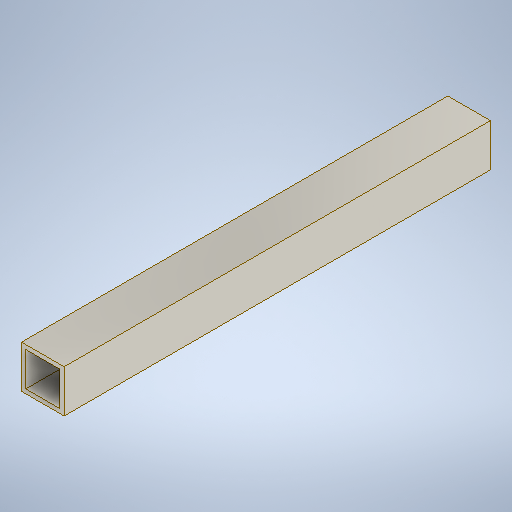
# Autodesk Inventor part: Sessao8_07_04_2025_0002_0001
Saved by Autodesk Inventor 2025.2 (Build 292293000, 293)
## iProperties
Created: 2025-04-07
Part Number: Sessao8_07_04_2025_0002_0001
Material: Titânio
Document SubType Name: Modeling
Designer: Gustavo Sousa
Density: 4.51 g/cm^3
Appearance: Titânio - Polido
Author: Gustavo Sousa
Autodesk Inventor part; units mm, degrees
ref_plane "YZ Plane" through (0, 0, 0) normal (1, 0, 0) x (0, 1, 0)
ref_plane "XZ Plane" through (0, 0, 0) normal (0, 1, 0) x (-1, 0, 0)
ref_plane "XY Plane" through (0, 0, 0) normal (0, 0, 1) x (1, 0, 0)
sketch "Esboço1" plane through (0, 0, 0) normal (0, 0, 1) x (1, 0, 0)
  line L0 (-10, -10) -> (10, -10)
  line L1 (10, -10) -> (10, 10)
  line L2 (10, 10) -> (-10, 10)
  line L3 (-10, 10) -> (-10, -10)
  line L4 (-10, -10) -> (10, 10) construction
  line L5 (10, -10) -> (-10, 10) construction
  line L6 (-8, -8) -> (8, -8)
  line L7 (8, -8) -> (8, 8)
  line L8 (8, 8) -> (-8, 8)
  line L9 (-8, 8) -> (-8, -8)
  line L10 (-8, -8) -> (8, 8) construction
  line L11 (8, -8) -> (-8, 8) construction
  point P0 (0, 0)
  dimension "d0" = 20
  dimension "d1" = 2
  constraints: 24 end point, 4 midpoint, 4 parallel, 4 perpendicular, 2 horizontal
  measures "d0" distance of L1.end L2.end
  measures "d1" distance between parallel lines of L2 L8
extrude "Extrusão1" add sketch "Esboço1" along normal mid plane 200
